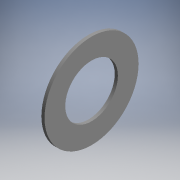
# Autodesk Inventor part: DIN-137 A 8
Saved by Autodesk Inventor 2017.3 (Build 213256000, 256)
## iProperties
Part Number: DIN-137 A 8
Material: Generic
Catalog Web Link: www.cadenas.de
Description: DIN-137 A-Wave spring washers
Vendor: FESTO
Document SubType Name: Modeling
Designer: partserver
Manufacturer: FESTO
Mass: 0.0606484 g
Surface Area: 2.7935 cm^2
Volume: 0.0606484 cm^3
Density: 1 g/cm^3
Appearance: PSOLRGB-175-175-175
Category: PARTsolutions
Company: FESTO
Title: Lock washer DIN 137 A 8
Author: Cadenas PARTsolutions
Comments: Wave spring washers
PSOL_IDENT_0: {$CADENAS_DATA\23d-libs\festo\zyl_zubeh\din_137a\din_137_a.prj},190 {VTYP=3D},{NB=DIN-137 A 8},{LINA=
PSOL_IDENT_1: Lock washer DIN 137 A 8},{NN=DIN-137 A},{DATE=28.05.2015 10:57:02},{GEOMDATE=13.03.2014 14:21:16},{V
PSOL_IDENT_2: ERSION=v130708133745},{LINEID=70},{WBVAR=},{WBNUMERIC=}  {NB=DIN-137 A 8},{LINA=Federscheibe DIN 137
PSOL_IDENT_3: A 8},{KT=X},{IDNR=},{NENN=A 8},{D=8.0},{DA=8.4},{DW=15.0},{H=0.50},{H1=3.400}
NB: DIN-137 A 8
NN: DIN-137 A
NT: Wave spring washers
NBSYN: DIN-137 $NENN.
LINA: Lock washer DIN 137 A 8
CATALOG: Festo
ROWDESC: A 8
OFFICIAL_STANDARD_NUMBERS: DIN 137
D: 8
DA: 8.4
DW: 15
H: 0.5
H1: 3.4
SUPPLIER: FESTO
ARTICLENO: DIN-137 A 8
BOMINFO: Lock washer DIN 137 A 8
CREATOR: CADENAS GmbH
Autodesk Inventor part; units mm, degrees
ref_plane "YZ Plane" through (0, 0, 0) normal (1, 0, 0) x (0, 1, 0)
ref_plane "XZ Plane" through (0, 0, 0) normal (0, 1, 0) x (-1, 0, 0)
ref_plane "XY Plane" through (0, 0, 0) normal (0, 0, 1) x (1, 0, 0)
sketch "Sketch_1" plane through (0, 0, 0) normal (1, 0, 0) x (0, 1, 0)
  circle A0 centre (0, 0) radius 7.5
  circle A1 centre (0, 0) radius 4.2
  constraints: 2 centre point
extrude "Extrusion1" add sketch "Sketch_1" along normal blind 0.5
ref_plane "IP1_XY" through (0, 0, 0) normal (1, 0, 0) x (0, 0, -1)
ref_plane "IP1_YZ" through (0, 0, 0) normal (0, 0, -1) x (0, 1, 0)
ref_plane "IP1_ZX" through (0, 0, 0) normal (0, 1, 0) x (1, 0, 0)
ref_plane "IP2_XY" through (0.5, 0, 0) normal (1, 0, 0) x (0, 0, -1)
ref_plane "IP2_YZ" through (0.5, 0, 0) normal (0, 0, -1) x (0, 1, 0)
ref_plane "IP2_ZX" through (0.5, 0, 0) normal (0, 1, 0) x (1, 0, 0)
body "Solid1"
